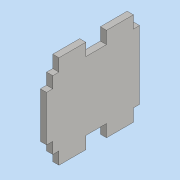
# Autodesk Inventor part: X-Motor-Housing_Motor-Side
Saved by Autodesk Inventor 2016 SP1 (Build 200210100, 210)
## iProperties
Created: 2016-02-22
Part Number: X-Motor-Housing_Motor-Side
Material: Generic
Document SubType Name: Modeling
Designer: Mohamed A.
Density: 1 g/cm^3
Appearance: Default
Author: Mohamed A.
Autodesk Inventor part; units mm, degrees
ref_plane "YZ Plane" through (0, 0, 0) normal (1, 0, 0) x (0, 1, 0)
ref_plane "XZ Plane" through (0, 0, 0) normal (0, 1, 0) x (-1, 0, 0)
ref_plane "XY Plane" through (0, 0, 0) normal (0, 0, 1) x (1, 0, 0)
sketch "Sketch2" plane through (0, 0, 0) normal (1, 0, 0) x (0, 1, 0)
  line L0 (21, -16.5) -> (18, -16.5)
  line L1 (-21, -16.5) -> (-21, -11)
  line L2 (-21, 16.5) -> (-18, 16.5)
  line L3 (21, 16.5) -> (21, -16.5)
  line L4 (21, -16.5) -> (-21, 16.5) construction
  line L5 (-21, -16.5) -> (21, 16.5) construction
  line L6 (0, -31.5) -> (0, 31.5) construction
  line L7 (-33, 0) -> (30, 0) construction
  line L8 (18, 16.5) -> (18, 22.5)
  line L9 (18, 22.5) -> (5, 22.5)
  line L10 (5, 22.5) -> (5, 16.5)
  line L11 (18, 16.5) -> (21, 16.5)
  line L12 (5, 16.5) -> (18, 16.5)
  line L13 (0, 16.5) -> (5, 16.5)
  line L14 (-18, 16.5) -> (-18, 22.5)
  line L15 (-18, 22.5) -> (-5, 22.5)
  line L16 (-5, 22.5) -> (-5, 16.5)
  line L17 (18, -16.5) -> (5, -16.5)
  line L18 (5, -16.5) -> (-5, -16.5)
  line L19 (-5, -16.5) -> (-18, -16.5)
  line L20 (-18, -16.5) -> (-21, -16.5)
  line L21 (-18, 16.5) -> (-5, 16.5)
  line L22 (-5, 16.5) -> (0, 16.5)
  line L23 (-21, 11) -> (-24, 11)
  line L24 (-24, 11) -> (-24, -11)
  line L25 (-24, -11) -> (-21, -11)
  line L26 (-21, 11) -> (-21, 16.5)
  line L27 (-21, -11) -> (-21, 11)
  line L28 (18, -16.5) -> (18, -22.5)
  line L29 (18, -22.5) -> (5, -22.5)
  line L30 (5, -22.5) -> (5, -16.5)
  line L31 (-5, -16.5) -> (-5, -22.5)
  line L32 (-5, -22.5) -> (-18, -22.5)
  line L33 (-18, -22.5) -> (-18, -16.5)
  point P0 (0, 0)
  dimension "d4" = 42
  dimension "d5" = 33
  dimension "d9" = 6
  dimension "d11" = 3
  dimension "d12" = 22
  dimension "d13" = 6
  dimension "d16" = 3
  dimension "d17" = 5
  constraints: 64 end point, 34 parallel, 29 perpendicular, 8 symmetric about line, 6 horizontal, 3 point on line, 2 midpoint, 2 vertical, 1 collinear
  measures "d4" distance of L2.start L3.start
  measures "d5" distance of L1.start L2.start
  measures "d9" distance of L8.start L8.end
  measures "d11" distance of L23.start L23.end
  measures "d12" distance between parallel lines of L25 L23
  measures "d13" distance of L0.end L28.end
  measures "d16" distance between parallel lines of L8 L3
  measures "d17" distance between parallel lines of L6 L10
extrude "Extrusion2" add sketch "Sketch2" against normal blind 3
equation "\"d12\" = 0.666667 * d5"
body "Solid2"
